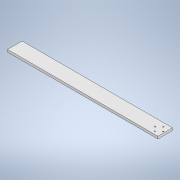
# Autodesk Inventor part: 横長2ndフラットバー
Saved by Autodesk Inventor 2022 (Build 260153000, 153)
## iProperties
Created: 2022-10-17
Part Number: 横長2ndフラットバー
Material: アルミニウム
Document SubType Name: Modeling
Designer: tdn82
Density: 2.7 g/cm^3
Appearance: サテン
Author: tdn82
Autodesk Inventor part; units mm, degrees
ref_plane "YZ Plane" through (0, 0, 0) normal (1, 0, 0) x (0, 1, 0)
ref_plane "XZ Plane" through (0, 0, 0) normal (0, 1, 0) x (-1, 0, 0)
ref_plane "XY Plane" through (0, 0, 0) normal (0, 0, 1) x (1, 0, 0)
sketch "スケッチ1" plane through (0, 0, 0) normal (1, 0, 0) x (0, 1, 0)
  line L0 (0, 0) -> (-5, 0)
  line L1 (-5, 0) -> (-5, -30)
  line L2 (-5, -30) -> (0, -30)
  line L3 (0, -30) -> (0, 0)
  dimension "d0" = 30
  dimension "d1" = 5
  constraints: 8 end point, 2 parallel, 1 horizontal, 1 perpendicular
  measures "d0" distance of L2.end L0.start
  measures "d1" distance of L0.start L0.end
extrude "押し出し1" add sketch "スケッチ1" along normal blind 310
sketch "スケッチ2" plane through (0, -5, -30) normal (0, -1, 0) x (1, 0, 0)
  line L0 (310, 30) -> (310, 0) projected
  line L1 (0, 0) -> (310, 0) projected
  point P0 (0, 30)
  point P1 (298.5, 16)
  dimension "d4" = 11.5
  dimension "d12" = 16
  measures "d4" distance from line of point (298.5, 16) L0
  measures "d12" distance from line of point (298.5, 16) L1
hole "穴1" at (298.5, -5, -14) direction (0, 1, 0) diameter 10 depth 1.5 tip angle 118
sketch "スケッチ3" plane through (0, -5, -30) normal (0, -1, 0) x (1, 0, 0)
  line L0 (310, 30) -> (310, 0) projected
  line L1 (310, 16) -> (272.6522, 16)
  line L2 (0, 0) -> (310, 0) projected
  circle A0 centre (298.5, 16) radius 5 projected
  point P0 (0, 30)
  point P1 (298.7741, 7.5)
  point P2 (307, 16.2741)
  point P3 (298.2259, 24.5)
  point P4 (290, 15.7259)
  dimension "d14" = 16
  dimension "d15" = 8.5
  dimension "d18" = 360
  constraints: 2 end point, 1 horizontal, 1 point on line, 5 other
  measures "d14" distance between parallel lines of L1 L2
  measures "d15" distance from line of point (298.774, 7.5) L1
hole "穴2" at (298.7741, -5, -22.5) at (307, -5, -13.7259) at (298.2259, -5, -5.5) at (290, -5, -14.2741) direction (0, 1, 0) diameter 2.5 end through all
